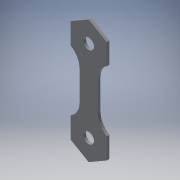
# Autodesk Inventor part: Leg
Saved by Autodesk Inventor 2016 (Build 200138000, 138)
## iProperties
Created: 2015-10-16
Part Number: Leg
Material: Generic
Document SubType Name: Modeling
Designer: powasar16
Density: 1 g/cm^3
Appearance: Default
Author: powasar16
Autodesk Inventor part; units mm, degrees
ref_plane "YZ Plane" through (0, 0, 0) normal (1, 0, 0) x (0, 1, 0)
ref_plane "XZ Plane" through (0, 0, 0) normal (0, 1, 0) x (-1, 0, 0)
ref_plane "XY Plane" through (0, 0, 0) normal (0, 0, 1) x (1, 0, 0)
sketch "Sketch1" plane through (0, 0, 0) normal (0, 0, 1) x (1, 0, 0)
  circle A0 centre (2.8854, -1.4956) radius 3.75 projected
  line L0 (2.8854, 13.1691) -> (15.5854, 5.8367)
  line L1 (15.5854, 5.8367) -> (15.5854, -8.828)
  line L2 (15.5854, -8.828) -> (2.8854, -16.1603) construction
  line L3 (2.8854, -16.1603) -> (-9.8146, -8.828) construction
  line L4 (-9.8146, -8.828) -> (-9.8146, 5.8367)
  line L5 (-9.8146, 5.8367) -> (2.8854, 13.1691)
  line L6 (-3.4646, -12.4941) -> (9.2354, -12.4941) construction
  line L7 (9.2354, -12.4941) -> (9.2354, -19.8265) construction
  line L8 (9.2354, -46.733) -> (-3.4646, -46.733) construction
  line L9 (-3.4646, -46.733) -> (-3.4646, -40.3147) construction
  line L10 (10.8229, -30.0706) -> (-5.0521, -30.0706) construction
  arc A1 (15.5854, -8.828) -> (9.2354, -19.8265) centre (21.9354, -19.8265) ccw
  line L11 (2.8854, -12.4941) -> (2.8854, -46.733) construction
  arc A2 (-3.4646, -19.8265) -> (-9.8146, -8.828) centre (-16.1646, -19.8265) ccw
  circle A3 centre (2.8854, -58.6456) radius 3.75
  line L12 (2.8854, -73.3103) -> (15.5854, -65.978)
  line L13 (15.5854, -65.978) -> (15.5854, -51.3133)
  line L14 (15.5854, -51.3133) -> (2.8854, -43.9809) construction
  line L15 (2.8854, -43.9809) -> (-9.8146, -51.3133) construction
  line L16 (-9.8146, -51.3133) -> (-9.8146, -65.978)
  line L17 (-9.8146, -65.978) -> (2.8854, -73.3103)
  arc A4 (9.2354, -40.3147) -> (15.5854, -51.3133) centre (21.9354, -40.3147) ccw
  arc A5 (-9.8146, -51.3133) -> (-3.4646, -40.3147) centre (-16.1646, -40.3147) ccw
  line L18 (9.2354, -19.8265) -> (9.2354, -40.3147)
  line L19 (-3.4646, -19.8265) -> (-3.4646, -12.4941) construction
  line L20 (-3.4646, -40.3147) -> (-3.4646, -19.8265)
  line L21 (9.2354, -40.3147) -> (9.2354, -46.733) construction
  point P0 (0, 0)
  dimension "d2" = 25.4
  dimension "d3" = 12.7
  dimension "d6" = 28.575
  dimension "d7" = 10.9985
  dimension "d8" = 11.9126
  constraints: 44 end point, 13 symmetric about line, 10 parallel, 8 point on circle, 4 centre point, 4 midpoint, 4 tangent, 3 perpendicular, 1 coincident, 1 horizontal, 17 other
  measures "d2" distance between parallel lines of L1 L4
  measures "d3" distance between parallel lines of L7 L9
  measures "d6" distance from line of A0.centre L10
  measures "d7" distance from line of A0.centre L6
  measures "d8" distance from line of L8 A3.centre
extrude "Extrusion1" add sketch "Sketch1" along normal blind 1.905
body "Solid1"
